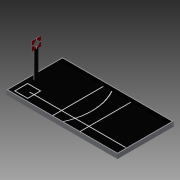
# Autodesk Inventor part: SEC 2014 Model1
Saved by Autodesk Inventor 2014 SP1 (Build 180222100, 222)
## iProperties
Created: 2014-01-13
Part Number: SEC 2014 Model1
Material: Generic
Document SubType Name: Modeling
Designer: Aaron
Density: 1 g/cm^3
Appearance: Default
Author: Aaron
Autodesk Inventor part; units mm, degrees
ref_plane "YZ Plane" through (0, 0, 0) normal (1, 0, 0) x (0, 1, 0)
ref_plane "XZ Plane" through (0, 0, 0) normal (0, 1, 0) x (-1, 0, 0)
ref_plane "XY Plane" through (0, 0, 0) normal (0, 0, 1) x (1, 0, 0)
sketch "Sketch1" plane through (0, 0, 0) normal (0, 1, 0) x (-1, 0, 0)
  line L0 (0, 0) -> (2463.8, 0)
  line L1 (2463.8, 0) -> (2463.8, -1244.6)
  line L2 (2463.8, -1244.6) -> (0, -1244.6)
  line L3 (0, -1244.6) -> (0, 0)
  dimension "d0" = 2463.8
  dimension "d1" = 1244.6
  constraints: 8 end point, 2 parallel, 1 horizontal, 1 perpendicular
  measures "d0" distance of L0.start L0.end
  measures "d1" distance of L2.end L0.start
extrude "Extrusion1" add sketch "Sketch1" along normal blind 12.7
sketch "Sketch2" plane through (0, 12.7, 0) normal (0, 1, 0) x (1, 0, 0)
  line L0 (-2463.8, 0) -> (0, 0) projected
  line L1 (0, 0) -> (0, 1244.6) projected
  line L2 (0, 1244.6) -> (-2463.8, 1244.6) projected
  line L3 (-2463.8, 1244.6) -> (-2463.8, 0) projected
  line L4 (-2444.75, 1225.55) -> (-19.05, 1225.55)
  line L5 (-19.05, 1225.55) -> (-19.05, 19.05)
  line L6 (-19.05, 19.05) -> (-2444.75, 19.05)
  line L7 (-2444.75, 19.05) -> (-2444.75, 1225.55)
  line L8 (-2463.8, 1244.6) -> (0, 1244.6)
  line L9 (0, 1244.6) -> (0, 0)
  line L10 (0, 0) -> (-2463.8, 0)
  line L11 (-2463.8, 0) -> (-2463.8, 1244.6)
  dimension "d4" = 19.05
  dimension "d5" = 19.05
  dimension "d6" = 19.05
  dimension "d7" = 19.05
  constraints: 16 end point, 4 parallel, 2 horizontal, 2 perpendicular
  measures "d4" distance from line of L2 L4.start
  measures "d5" distance from line of L3 L4.start
  measures "d6" distance from line of L1 L5.end
  measures "d7" distance from line of L0 L5.end
extrude "Extrusion2" add sketch "Sketch2" along normal blind 88.9
sketch "Sketch3" plane through (0, 12.7, 0) normal (0, 1, 0) x (1, 0, 0)
  line L0 (-19.05, 1225.55) -> (-2444.75, 1225.55) projected
  line L1 (-19.05, 19.05) -> (-19.05, 1225.55) projected
  line L2 (-19.05, 1225.55) -> (-2444.75, 1225.55) projected
  line L3 (-2444.75, 1225.55) -> (-2444.75, 19.05) projected
  line L4 (-2444.75, 19.05) -> (-19.05, 19.05) projected
  line L5 (-2463.8, 0) -> (0, 0) projected
  line L6 (-2463.8, 1244.6) -> (-2463.8, 0) projected
  line L7 (-19.05, 19.05) -> (-2444.75, 19.05) projected
  line L8 (-2444.75, 146.05) -> (-2139.95, 146.05)
  line L9 (-2139.95, 146.05) -> (-2139.95, 450.85)
  line L10 (-2139.95, 450.85) -> (-2444.75, 450.85)
  line L11 (-2444.75, 450.85) -> (-2444.75, 146.05)
  line L12 (-2425.7, 431.8) -> (-2159, 431.8)
  line L13 (-2159, 431.8) -> (-2159, 165.1)
  line L14 (-2159, 165.1) -> (-2425.7, 165.1)
  line L15 (-2425.7, 165.1) -> (-2425.7, 431.8)
  line L16 (-2248.2339, 307.975) -> (-114.6339, 307.975)
  line L17 (-114.6339, 307.975) -> (-114.6339, 288.925)
  line L18 (-114.6339, 288.925) -> (-2248.2339, 288.925)
  line L19 (-2248.2339, 288.925) -> (-2248.2339, 307.975)
  line L20 (-1549.4, 1225.55) -> (-1530.35, 1225.55)
  line L21 (-1530.35, 1225.55) -> (-1530.35, 19.05)
  line L22 (-1530.35, 19.05) -> (-1549.4, 19.05)
  line L23 (-1549.4, 19.05) -> (-1549.4, 1225.55)
  line L24 (-939.8, 1225.55) -> (-920.75, 1225.55)
  line L25 (-920.75, 1225.55) -> (-920.75, 19.05)
  line L26 (-920.75, 19.05) -> (-939.8, 19.05)
  line L27 (-939.8, 19.05) -> (-939.8, 1225.55)
  line L28 (-2444.75, 666.75) -> (-2425.7, 666.75)
  line L29 (-2425.7, 666.75) -> (-2425.7, 577.85)
  line L30 (-2425.7, 577.85) -> (-2444.75, 577.85)
  line L31 (-2444.75, 577.85) -> (-2444.75, 666.75)
  arc A0 (-1352.0706, 0) -> (-1341.2523, 1225.55) centre (-2425.7, 622.3) ccw
  arc A1 (-1374.1473, 0) -> (-1363.1042, 1225.55) centre (-2425.7, 622.3) ccw
  arc A2 (-1363.0943, 0) -> (-1352.1649, 19.05) centre (-2425.7, 622.3) ccw
  arc A3 (-1240.2679, 288.925) -> (-1235.075, 307.975) centre (-2425.7, 622.3) ccw
  line L32 (-1363.1042, 1225.55) -> (-1341.2523, 1225.55)
  line L33 (-1341.2523, 19.05) -> (-1363.1042, 19.05)
  point P0 (-2248.2339, 298.45)
  point P1 (-2444.75, 622.3)
  dimension "d10" = 127
  dimension "d11" = 304.8
  dimension "d12" = 304.8
  dimension "d13" = 19.05
  dimension "d14" = 19.05
  dimension "d15" = 266.7
  dimension "d16" = 266.7
  dimension "d17" = 9.525
  dimension "d18" = 2133.6
  dimension "d19" = 19.05
  dimension "d20" = 609.6
  dimension "d21" = 19.05
  dimension "d22" = 609.6
  dimension "d23" = 19.05
  dimension "d24" = 295.275
  dimension "d25" = 603.25
  dimension "d26" = 44.45
  dimension "d27" = 88.9
  dimension "d28" = 19.05
  dimension "d30" = 2481.8842
  dimension "d31" = 2443.7842
  constraints: 52 end point, 12 parallel, 11 point on line, 10 point on circle, 6 horizontal, 6 perpendicular, 4 centre point, 4 coincident, 2 midpoint, 1 collinear, 6 other
  measures "d10" distance of point (-2444.75, 19.05) L8.start
  measures "d11" distance of L8.start L8.end
  measures "d12" distance of L8.end L9.end
  measures "d13" distance from line of L10 L12.start
  measures "d14" distance from line of L11 L12.start
  measures "d15" distance of L12.start L12.end
  measures "d16" distance of L14.end L12.start
  measures "d17" distance of L16.start point (-2248.234, 298.45)
  measures "d18" distance of L16.start L16.end
  measures "d19" distance of L18.end L16.start
  measures "d20" distance from line of L13 L20.start
  measures "d21" distance between parallel lines of L21 L23
  measures "d22" distance of L24.start L20.start
  measures "d23" distance between parallel lines of L25 L27
  measures "d24" distance from line of A3.end L21
  measures "d25" distance from line of L0 point (-2444.75, 622.3)
  measures "d26" distance of point (-2444.75, 622.3) L28.start
  measures "d27" distance of L28.end L29.end
  measures "d28" distance of L28.start L28.end
  measures "d30" diameter of A0
  measures "d31" diameter of A1
extrude "Extrusion3" add sketch "Sketch3" along normal blind 1.5875 contours L25 L16 L27 L0 | L25 L18 L27 L16 | L16 L17 L18 L25 | L4 L27 L18 L25 | A0 L16 A1 L0 | L27 L18 A0 L16 | A0 L18 A3 L16 | L4 A1 L18 A0 | L21 L16 L23 L0 | A1 L18 L21 L16 | L16 A3 L18 A1 | A2 L5 A1 L4 | L21 L18 L23 L16 | L23 L18 L9 L16 | L21 L4 L23 L18 | L28 L29 L30 L3 | L16 L13 L12 L15 L14 L18 L9 L8 L3 L10 | L9 L18 L13 L16 | L13 L18 L19 L16
sketch "Sketch4" plane through (0, 12.7, 0) normal (0, 1, 0) x (1, 0, 0)
  line L0 (-1363.1042, 1225.55) -> (-1530.35, 1225.55) projected
  line L1 (-1530.35, 1225.55) -> (-1530.35, 307.975) projected
  line L2 (-2444.75, 1225.55) -> (-19.05, 1225.55) projected
  circle A0 centre (-1564.3323, 1073.15) radius 3.175
  circle A1 centre (-1564.3323, 1022.35) radius 3.175
  circle A2 centre (-1564.3323, 971.55) radius 3.175
  circle A3 centre (-1564.3323, 920.75) radius 3.175
  circle A4 centre (-1564.3323, 869.95) radius 3.175
  circle A5 centre (-1564.3323, 819.15) radius 3.175
  circle A6 centre (-1564.3323, 768.35) radius 3.175
  circle A7 centre (-1564.3323, 717.55) radius 3.175
  circle A8 centre (-1564.3323, 666.75) radius 3.175
  circle A9 centre (-1564.3323, 615.95) radius 3.175
  circle A10 centre (-1564.3323, 565.15) radius 3.175
  circle A11 centre (-1564.3323, 514.35) radius 3.175
  circle A12 centre (-1564.3323, 463.55) radius 3.175
  circle A13 centre (-1564.3323, 412.75) radius 3.175
  circle A14 centre (-1513.5323, 1073.15) radius 3.175
  circle A15 centre (-1513.5323, 1022.35) radius 3.175
  circle A16 centre (-1513.5323, 971.55) radius 3.175
  circle A17 centre (-1513.5323, 920.75) radius 3.175
  circle A18 centre (-1513.5323, 869.95) radius 3.175
  circle A19 centre (-1513.5323, 819.15) radius 3.175
  circle A20 centre (-1513.5323, 768.35) radius 3.175
  circle A21 centre (-1513.5323, 717.55) radius 3.175
  circle A22 centre (-1513.5323, 666.75) radius 3.175
  circle A23 centre (-1513.5323, 615.95) radius 3.175
  circle A24 centre (-1513.5323, 565.15) radius 3.175
  circle A25 centre (-1513.5323, 514.35) radius 3.175
  circle A26 centre (-1513.5323, 463.55) radius 3.175
  circle A27 centre (-1513.5323, 412.75) radius 3.175
  point P0 (0, 0)
  point P1 (-1353.5792, 1225.55)
  point P2 (-1378.9792, 1225.55)
  dimension "d38" = 152.4
  dimension "d41" = 50.8
  dimension "d42" = 6.35
  dimension "d45" = 50.8
  dimension "d50" = 6.35
  dimension "d53" = 50.8
  dimension "d58" = 9.525
  dimension "d59" = 25.4
  constraints: 28 centre point, 3 coincident, 2 point on line, 2 vertical, 52 other
  measures "d38" distance from line of L0 point (-1513.532, 1073.15)
  measures "d41" distance of point (-1564.332, 1073.15) point (-1564.332, 1022.35)
  measures "d42" diameter of A0
  measures "d45" distance of A0.centre A1.centre
  measures "d50" diameter of A14
  measures "d53" distance of A14.centre A15.centre
  measures "d58" distance of point (-1363.104, 1225.55) point (-1353.579, 1225.55)
  measures "d59" distance of point (-1353.579, 1225.55) point (-1378.979, 1225.55)
extrude "Extrusion4" cut sketch "Sketch4" against normal blind 25.4
sketch "Sketch5" plane through (0, 12.7, 0) normal (0, 1, 0) x (1, 0, 0)
  arc A0 (-1225.2263, 307.975) -> (-1341.2523, 1225.55) centre (-2425.7, 622.3) ccw projected
  line L0 (-1225.2263, 307.975) -> (-939.8, 307.975) projected
  line L1 (-939.8, 307.975) -> (-939.8, 1225.55) projected
  line L2 (-939.8, 1225.55) -> (-1341.2523, 1225.55) projected
  line L3 (-920.75, 1225.55) -> (-920.75, 307.975) projected
  line L4 (-920.75, 307.975) -> (-114.6339, 307.975) projected
  line L5 (-114.6339, 307.975) -> (-114.6339, 288.925) projected
  line L6 (-114.6339, 288.925) -> (-920.75, 288.925) projected
  line L7 (-920.75, 288.925) -> (-920.75, 19.05) projected
  line L8 (-920.75, 19.05) -> (-19.05, 19.05) projected
  line L9 (-19.05, 19.05) -> (-19.05, 1225.55) projected
  line L10 (-19.05, 1225.55) -> (-920.75, 1225.55) projected
  line L11 (-1341.2523, 19.05) -> (-1363.1042, 19.05) projected
  arc A1 (-1341.2523, 19.05) -> (-1230.3764, 288.925) centre (-2425.7, 622.3) ccw projected
  line L12 (-1230.3764, 288.925) -> (-939.8, 288.925) projected
  line L13 (-939.8, 288.925) -> (-939.8, 19.05) projected
  line L14 (-920.75, 19.05) -> (-939.8, 19.05) projected
  line L15 (-920.75, 19.05) -> (-920.75, 288.925) projected
  line L16 (-920.75, 288.925) -> (-114.6339, 288.925) projected
  line L17 (-114.6339, 288.925) -> (-114.6339, 307.975) projected
  line L18 (-114.6339, 307.975) -> (-920.75, 307.975) projected
  line L19 (-920.75, 307.975) -> (-920.75, 1225.55) projected
  line L20 (-939.8, 1225.55) -> (-920.75, 1225.55) projected
  line L21 (-939.8, 1225.55) -> (-939.8, 307.975) projected
  line L22 (-939.8, 307.975) -> (-1225.2263, 307.975) projected
  arc A2 (-1225.2263, 307.975) -> (-1341.2523, 1225.55) centre (-2425.7, 622.3) ccw projected
  line L23 (-1363.1042, 1225.55) -> (-1341.2523, 1225.55) projected
  arc A3 (-1244.929, 307.975) -> (-1363.1042, 1225.55) centre (-2425.7, 622.3) ccw projected
  line L24 (-1244.929, 307.975) -> (-1530.35, 307.975) projected
  line L25 (-1530.35, 307.975) -> (-1530.35, 1225.55) projected
  line L26 (-1549.4, 1225.55) -> (-1530.35, 1225.55) projected
  line L27 (-1549.4, 1225.55) -> (-1549.4, 307.975) projected
  line L28 (-1549.4, 307.975) -> (-2139.95, 307.975) projected
  line L29 (-2139.95, 307.975) -> (-2139.95, 450.85) projected
  line L30 (-2139.95, 450.85) -> (-2444.75, 450.85) projected
  line L31 (-2444.75, 146.05) -> (-2444.75, 450.85) projected
  line L32 (-2444.75, 146.05) -> (-2139.95, 146.05) projected
  line L33 (-2139.95, 146.05) -> (-2139.95, 288.925) projected
  line L34 (-2139.95, 288.925) -> (-1549.4, 288.925) projected
  line L35 (-1549.4, 288.925) -> (-1549.4, 19.05) projected
  line L36 (-1530.35, 19.05) -> (-1549.4, 19.05) projected
  line L37 (-1530.35, 19.05) -> (-1530.35, 288.925) projected
  line L38 (-1530.35, 288.925) -> (-1250.1655, 288.925) projected
  arc A4 (-1363.1042, 19.05) -> (-1250.1655, 288.925) centre (-2425.7, 622.3) ccw projected
  line L39 (-2159, 288.925) -> (-2159, 165.1) projected
  line L40 (-2159, 165.1) -> (-2425.7, 165.1) projected
  line L41 (-2425.7, 165.1) -> (-2425.7, 431.8) projected
  line L42 (-2425.7, 431.8) -> (-2159, 431.8) projected
  line L43 (-2159, 431.8) -> (-2159, 307.975) projected
  line L44 (-2159, 307.975) -> (-2248.2339, 307.975) projected
  line L45 (-2248.2339, 307.975) -> (-2248.2339, 288.925) projected
  line L46 (-2248.2339, 288.925) -> (-2159, 288.925) projected
  line L47 (-19.05, 1225.55) -> (-19.05, 19.05) projected
  line L48 (-19.05, 19.05) -> (-2444.75, 19.05) projected
  line L49 (-2444.75, 19.05) -> (-2444.75, 1225.55) projected
  line L50 (-2444.75, 1225.55) -> (-19.05, 1225.55) projected
  line L51 (0, 0) -> (0, 1244.6) projected
  line L52 (0, 1244.6) -> (-2463.8, 1244.6) projected
  line L53 (-2463.8, 1244.6) -> (-2463.8, 0) projected
  line L54 (-2463.8, 0) -> (0, 0) projected
  line L55 (-2444.75, 1225.55) -> (-19.05, 1225.55) projected
  arc A5 (-1352.1649, 19.05) -> (-1352.1649, 1225.55) centre (-2425.7, 622.3) ccw
  circle A6 centre (-1305.1845, 1073.15) radius 3.175
  circle A7 centre (-1286.4764, 1022.35) radius 3.175
  circle A8 centre (-1235.6764, 1022.35) radius 3.175
  circle A9 centre (-1270.2475, 971.55) radius 3.175
  circle A10 centre (-1219.4475, 971.55) radius 3.175
  circle A11 centre (-1256.3968, 920.75) radius 3.175
  circle A12 centre (-1205.5968, 920.75) radius 3.175
  circle A13 centre (-1244.8423, 869.95) radius 3.175
  circle A14 centre (-1194.0423, 869.95) radius 3.175
  circle A15 centre (-1235.5186, 819.15) radius 3.175
  circle A16 centre (-1184.7186, 819.15) radius 3.175
  circle A17 centre (-1254.3845, 1073.15) radius 3.175
  circle A18 centre (-1228.3746, 768.35) radius 3.175
  circle A19 centre (-1177.5746, 768.35) radius 3.175
  circle A20 centre (-1223.3722, 717.55) radius 3.175
  circle A21 centre (-1172.5722, 717.55) radius 3.175
  circle A22 centre (-1220.4854, 666.75) radius 3.175
  circle A23 centre (-1169.6854, 666.75) radius 3.175
  circle A24 centre (-1219.6993, 615.95) radius 3.175
  circle A25 centre (-1168.8993, 615.95) radius 3.175
  circle A26 centre (-1221.0098, 565.15) radius 3.175
  circle A27 centre (-1170.2098, 565.15) radius 3.175
  circle A28 centre (-1224.4236, 514.35) radius 3.175
  circle A29 centre (-1173.6236, 514.35) radius 3.175
  circle A30 centre (-1229.9585, 463.55) radius 3.175
  circle A31 centre (-1179.1585, 463.55) radius 3.175
  circle A32 centre (-1237.6434, 412.75) radius 3.175
  circle A33 centre (-1186.8434, 412.75) radius 3.175
  point P0 (-1279.7845, 1073.15)
  point P1 (-1261.0764, 1022.35)
  point P2 (-1244.8475, 971.55)
  point P3 (-1230.9968, 920.75)
  point P4 (-1219.4423, 869.95)
  point P5 (-1210.1186, 819.15)
  point P6 (-1202.9746, 768.35)
  point P7 (-1197.9722, 717.55)
  point P8 (-1195.0854, 666.75)
  point P9 (-1195.0854, 666.75)
  point P10 (-1194.2993, 615.95)
  point P11 (-1195.6098, 565.15)
  point P12 (-1199.0236, 514.35)
  point P13 (-1204.5585, 463.55)
  point P14 (-1212.2434, 412.75)
  point P15 (-1230.9968, 920.75)
  point P16 (-1219.4423, 869.95)
  dimension "d62" = 2462.8342
  dimension "d63" = 152.4
  dimension "d64" = 25.4
  dimension "d65" = 25.4
  dimension "d67" = 6.35
  dimension "d68" = 203.2
  dimension "d69" = 25.4
  dimension "d70" = 25.4
  dimension "d71" = 50.8
  dimension "d72" = 25.4
  dimension "d73" = 25.4
  dimension "d74" = 50.8
  dimension "d75" = 50.8
  dimension "d76" = 50.8
  dimension "d77" = 50.8
  dimension "d78" = 50.8
  dimension "d79" = 50.8
  dimension "d80" = 50.8
  dimension "d81" = 50.8
  dimension "d82" = 50.8
  dimension "d83" = 50.8
  dimension "d84" = 50.8
  dimension "d85" = 25.4
  dimension "d86" = 25.4
  dimension "d87" = 25.4
  dimension "d88" = 25.4
  dimension "d89" = 25.4
  dimension "d90" = 25.4
  dimension "d91" = 25.4
  dimension "d92" = 25.4
  dimension "d93" = 25.4
  dimension "d94" = 25.4
  dimension "d95" = 25.4
  dimension "d96" = 25.4
  dimension "d97" = 25.4
  dimension "d98" = 25.4
  dimension "d99" = 25.4
  dimension "d100" = 25.4
  dimension "d101" = 25.4
  dimension "d102" = 25.4
  dimension "d103" = 25.4
  dimension "d104" = 25.4
  dimension "d105" = 25.4
  dimension "d106" = 25.4
  dimension "d107" = 6.35
  dimension "d108" = 6.35
  dimension "d109" = 6.35
  dimension "d110" = 6.35
  dimension "d111" = 6.35
  dimension "d112" = 6.35
  dimension "d113" = 6.35
  dimension "d114" = 6.35
  dimension "d115" = 6.35
  dimension "d116" = 6.35
  dimension "d117" = 6.35
  dimension "d118" = 6.35
  dimension "d119" = 6.35
  dimension "d120" = 6.35
  dimension "d121" = 6.35
  dimension "d122" = 6.35
  dimension "d123" = 6.35
  dimension "d124" = 6.35
  dimension "d125" = 6.35
  dimension "d126" = 6.35
  dimension "d127" = 6.35
  constraints: 31 coincident, 28 centre point, 1 point on line, 21 other
  measures "d64" distance of point (-1305.184, 1073.15) point (-1279.784, 1073.15)
  measures "d65" distance of point (-1254.384, 1073.15) point (-1279.784, 1073.15)
  measures "d67" diameter of A6
  measures "d68" distance from line of L2 point (-1261.076, 1022.35)
  measures "d69" distance of point (-1261.076, 1022.35) point (-1286.476, 1022.35)
  measures "d70" distance of point (-1235.676, 1022.35) point (-1261.076, 1022.35)
  measures "d71" vertical distance of point (-1261.076, 1022.35) point (-1244.848, 971.55)
  measures "d72" distance of point (-1244.848, 971.55) point (-1270.248, 971.55)
  measures "d73" distance of point (-1244.848, 971.55) point (-1219.448, 971.55)
  measures "d74" vertical distance of point (-1244.848, 971.55) point (-1230.997, 920.75)
  measures "d75" vertical distance of point (-1230.997, 920.75) point (-1219.442, 869.95)
  measures "d76" vertical distance of point (-1219.442, 869.95) point (-1210.119, 819.15)
  measures "d77" vertical distance of point (-1202.975, 768.35) point (-1210.119, 819.15)
  measures "d78" vertical distance of point (-1202.975, 768.35) point (-1197.972, 717.55)
  measures "d79" vertical distance of point (-1197.972, 717.55) point (-1195.085, 666.75)
  measures "d80" vertical distance of point (-1195.085, 666.75) point (-1194.299, 615.95)
  measures "d81" vertical distance of point (-1194.299, 615.95) point (-1195.61, 565.15)
  measures "d82" vertical distance of point (-1195.61, 565.15) point (-1199.024, 514.35)
  measures "d83" vertical distance of point (-1199.024, 514.35) point (-1204.559, 463.55)
  measures "d84" vertical distance of point (-1212.243, 412.75) point (-1204.559, 463.55)
  measures "d85" distance of point (-1256.397, 920.75) point (-1230.997, 920.75)
  measures "d86" distance of point (-1205.597, 920.75) point (-1230.997, 920.75)
  measures "d87" distance of point (-1219.442, 869.95) point (-1244.842, 869.95)
  measures "d88" distance of point (-1194.042, 869.95) point (-1219.442, 869.95)
  measures "d89" distance of point (-1210.119, 819.15) point (-1235.519, 819.15)
  measures "d90" distance of point (-1184.719, 819.15) point (-1210.119, 819.15)
  measures "d91" distance of point (-1202.975, 768.35) point (-1228.375, 768.35)
  measures "d92" distance of point (-1177.575, 768.35) point (-1202.975, 768.35)
  measures "d93" distance of point (-1197.972, 717.55) point (-1223.372, 717.55)
  measures "d94" distance of point (-1172.572, 717.55) point (-1197.972, 717.55)
  measures "d95" distance of point (-1195.085, 666.75) point (-1220.485, 666.75)
  measures "d96" distance of point (-1169.685, 666.75) point (-1195.085, 666.75)
  measures "d97" distance of point (-1194.299, 615.95) point (-1219.699, 615.95)
  measures "d98" distance of point (-1168.899, 615.95) point (-1194.299, 615.95)
  measures "d99" distance of point (-1195.61, 565.15) point (-1221.01, 565.15)
  measures "d100" distance of point (-1170.21, 565.15) point (-1195.61, 565.15)
  measures "d101" distance of point (-1199.024, 514.35) point (-1224.424, 514.35)
  measures "d102" distance of point (-1173.624, 514.35) point (-1199.024, 514.35)
  measures "d103" distance of point (-1179.159, 463.55) point (-1204.559, 463.55)
  measures "d104" distance of point (-1204.559, 463.55) point (-1229.959, 463.55)
  measures "d105" distance of point (-1212.243, 412.75) point (-1237.643, 412.75)
  measures "d106" distance of point (-1186.843, 412.75) point (-1212.243, 412.75)
  measures "d107" diameter of A7
  measures "d108" diameter of A8
  measures "d109" diameter of A9
  measures "d110" diameter of A10
  measures "d111" diameter of A11
  measures "d112" diameter of A12
  measures "d113" diameter of A13
  measures "d114" diameter of A14
  measures "d115" diameter of A15
  measures "d116" diameter of A16
  measures "d117" diameter of A17
  measures "d118" diameter of A18
  measures "d119" diameter of A19
  measures "d120" diameter of A20
  measures "d121" diameter of A21
  measures "d122" diameter of A22
  measures "d123" diameter of A23
  measures "d124" diameter of A24
  measures "d125" diameter of A25
  measures "d126" diameter of A26
  measures "d127" diameter of A27
extrude "Extrusion5" cut sketch "Sketch5" against normal blind 25.4 contours A6 | A7 | A8 | A9 | A10 | A11 | A12 | A13 | A14 | A15 | A16 | A17 | A18 | A19 | A20 | A21 | A22 | A23 | A24 | A25 | A26 | A27 | A28 | A29 | A30 | A31 | A32 | A33
sketch "Sketch6" plane through (0, 12.7, 0) normal (0, 1, 0) x (1, 0, 0)
  line L0 (-939.8, 1225.55) -> (-939.8, 307.975) projected
  circle A0 centre (-1229.9585, 463.55) radius 3.175 projected
  circle A1 centre (-1221.0098, 565.15) radius 3.175 projected
  circle A2 centre (-1220.4854, 666.75) radius 3.175 projected
  circle A3 centre (-1228.3746, 768.35) radius 3.175 projected
  circle A4 centre (-1244.8423, 869.95) radius 3.175 projected
  circle A5 centre (-1270.2475, 971.55) radius 3.175 projected
  circle A6 centre (-1305.1845, 1073.15) radius 3.175 projected
  circle A7 centre (-1179.1585, 463.55) radius 3.175 projected
  circle A8 centre (-1170.2098, 565.15) radius 3.175 projected
  circle A9 centre (-1169.6854, 666.75) radius 3.175 projected
  circle A10 centre (-1177.5746, 768.35) radius 3.175 projected
  circle A11 centre (-1184.7186, 819.15) radius 3.175 projected
  circle A12 centre (-1205.5968, 920.75) radius 3.175 projected
  circle A13 centre (-1235.6764, 1022.35) radius 3.175 projected
  circle A14 centre (-1219.4475, 971.55) radius 3.175 projected
  circle A15 centre (-1194.0423, 869.95) radius 3.175 projected
  circle A16 centre (-1254.3845, 1073.15) radius 3.175 projected
  circle A17 centre (-1172.5722, 717.55) radius 3.175 projected
  circle A18 centre (-1168.8993, 615.95) radius 3.175 projected
  circle A19 centre (-1173.6236, 514.35) radius 3.175 projected
  circle A20 centre (-1186.8434, 412.75) radius 3.175 projected
  circle A21 centre (-1286.4764, 1022.35) radius 3.175 projected
  circle A22 centre (-1256.3968, 920.75) radius 3.175 projected
  circle A23 centre (-1235.5186, 819.15) radius 3.175 projected
  circle A24 centre (-1223.3722, 717.55) radius 3.175 projected
  circle A25 centre (-1219.6993, 615.95) radius 3.175 projected
  circle A26 centre (-1224.4236, 514.35) radius 3.175 projected
  circle A27 centre (-1237.6434, 412.75) radius 3.175 projected
  circle A28 centre (-1513.5323, 463.55) radius 3.175 projected
  circle A29 centre (-1513.5323, 565.15) radius 3.175 projected
  circle A30 centre (-1513.5323, 666.75) radius 3.175 projected
  circle A31 centre (-1513.5323, 768.35) radius 3.175 projected
  circle A32 centre (-1513.5323, 869.95) radius 3.175 projected
  circle A33 centre (-1513.5323, 971.55) radius 3.175 projected
  circle A34 centre (-1513.5323, 1073.15) radius 3.175 projected
  circle A35 centre (-1564.3323, 463.55) radius 3.175 projected
  circle A36 centre (-1564.3323, 565.15) radius 3.175 projected
  circle A37 centre (-1564.3323, 666.75) radius 3.175 projected
  circle A38 centre (-1564.3323, 768.35) radius 3.175 projected
  circle A39 centre (-1564.3323, 869.95) radius 3.175 projected
  circle A40 centre (-1564.3323, 971.55) radius 3.175 projected
  circle A41 centre (-1564.3323, 1073.15) radius 3.175 projected
  circle A42 centre (-1564.3323, 1022.35) radius 3.175 projected
  circle A43 centre (-1564.3323, 920.75) radius 3.175 projected
  circle A44 centre (-1564.3323, 819.15) radius 3.175 projected
  circle A45 centre (-1564.3323, 717.55) radius 3.175 projected
  circle A46 centre (-1564.3323, 615.95) radius 3.175 projected
  circle A47 centre (-1564.3323, 514.35) radius 3.175 projected
  circle A48 centre (-1564.3323, 412.75) radius 3.175 projected
  circle A49 centre (-1513.5323, 1022.35) radius 3.175 projected
  circle A50 centre (-1513.5323, 920.75) radius 3.175 projected
  circle A51 centre (-1513.5323, 819.15) radius 3.175 projected
  circle A52 centre (-1513.5323, 717.55) radius 3.175 projected
  circle A53 centre (-1513.5323, 615.95) radius 3.175 projected
  circle A54 centre (-1513.5323, 514.35) radius 3.175 projected
  circle A55 centre (-1513.5323, 412.75) radius 3.175 projected
  line L1 (0, 0) -> (-2463.8, 0) projected
  line L2 (-2463.8, 0) -> (-2463.8, 1244.6) projected
  line L3 (-2463.8, 1244.6) -> (0, 1244.6) projected
  line L4 (0, 1244.6) -> (0, 0) projected
  circle A56 centre (-955.675, 1073.15) radius 3.175
  circle A57 centre (-904.875, 1073.15) radius 3.175
  circle A58 centre (-955.675, 1022.35) radius 3.175
  circle A59 centre (-904.875, 1022.35) radius 3.175
  circle A60 centre (-955.675, 971.55) radius 3.175
  circle A61 centre (-904.875, 971.55) radius 3.175
  circle A62 centre (-955.675, 920.75) radius 3.175
  circle A63 centre (-904.875, 920.75) radius 3.175
  circle A64 centre (-955.675, 869.95) radius 3.175
  circle A65 centre (-904.875, 869.95) radius 3.175
  circle A66 centre (-955.675, 819.15) radius 3.175
  circle A67 centre (-904.875, 819.15) radius 3.175
  circle A68 centre (-955.675, 768.35) radius 3.175
  circle A69 centre (-904.875, 768.35) radius 3.175
  circle A70 centre (-955.675, 717.55) radius 3.175
  circle A71 centre (-904.875, 717.55) radius 3.175
  circle A72 centre (-955.675, 666.75) radius 3.175
  circle A73 centre (-904.875, 666.75) radius 3.175
  circle A74 centre (-955.675, 615.95) radius 3.175
  circle A75 centre (-904.875, 615.95) radius 3.175
  circle A76 centre (-955.675, 565.15) radius 3.175
  circle A77 centre (-904.875, 565.15) radius 3.175
  circle A78 centre (-955.675, 514.35) radius 3.175
  circle A79 centre (-904.875, 514.35) radius 3.175
  circle A80 centre (-955.675, 463.55) radius 3.175
  circle A81 centre (-904.875, 463.55) radius 3.175
  circle A82 centre (-955.675, 412.75) radius 3.175
  circle A83 centre (-904.875, 412.75) radius 3.175
  point P0 (-920.75, 1225.55)
  point P1 (-930.275, 1225.55)
  point P2 (-930.275, 1073.15)
  dimension "d136" = 9.525
  dimension "d137" = 152.4
  dimension "d138" = 25.4
  dimension "d139" = 25.4
  dimension "d140" = 6.35
  dimension "d141" = 6.35
  dimension "d144" = 50.8
  constraints: 28 centre point, 2 coincident, 1 vertical, 52 other
  measures "d136" distance of point (-920.75, 1225.55) point (-930.275, 1225.55)
  measures "d137" distance of point (-930.275, 1225.55) point (-930.275, 1073.15)
  measures "d138" distance of point (-955.675, 1073.15) point (-930.275, 1073.15)
  measures "d139" distance of point (-904.875, 1073.15) point (-930.275, 1073.15)
  measures "d140" diameter of A56
  measures "d141" diameter of A57
  measures "d144" distance of A56.centre A58.centre
extrude "Extrusion6" cut sketch "Sketch6" against normal blind 25.4 contours A56 | A57 | A58 | A59 | A60 | A61 | A62 | A63 | A64 | A65 | A66 | A67 | A68 | A69 | A70 | A71 | A72 | A73 | A74 | A75 | A76 | A77 | A78 | A79 | A80 | A81 | A82 | A83
sketch "Sketch7" plane through (0, 14.2875, 0) normal (0, 1, 0) x (1, 0, 0)
  line L0 (-2444.75, 577.85) -> (-2444.75, 666.75) projected
  line L1 (-2444.75, 577.85) -> (-2425.7, 577.85) projected
  line L2 (-2444.75, 666.75) -> (-2425.7, 666.75)
  line L3 (-2425.7, 666.75) -> (-2425.7, 577.85)
  line L4 (-2425.7, 577.85) -> (-2444.75, 577.85)
  line L5 (-2444.75, 577.85) -> (-2444.75, 666.75)
  point P0 (0, 0)
  constraints: 8 end point, 2 parallel, 1 horizontal, 1 perpendicular
extrude "Extrusion7" add sketch "Sketch7" along normal blind 608.0125
sketch "Sketch8" plane through (-2425.7, 12.7, -577.85) normal (1, 0, 0) x (0, 0, -1)
  line L0 (0, 609.6) -> (88.9, 609.6) projected
  line L1 (-57.15, 584.2) -> (146.05, 584.2)
  line L2 (146.05, 584.2) -> (146.05, 787.4)
  line L3 (146.05, 787.4) -> (-57.15, 787.4)
  line L4 (-57.15, 787.4) -> (-57.15, 584.2)
  point P0 (-577.85, -12.7)
  point P1 (44.45, 584.2)
  dimension "d153" = 25.4
  dimension "d154" = 101.6
  dimension "d155" = 203.2
  dimension "d156" = 203.2
  constraints: 8 end point, 2 parallel, 1 horizontal, 1 perpendicular
  measures "d153" distance from line of L0 point (44.45, 584.2)
  measures "d154" distance of L1.start point (44.45, 584.2)
  measures "d155" distance of L3.end L1.start
  measures "d156" distance of L2.end L3.end
extrude "Extrusion8" add sketch "Sketch8" along normal blind 6.35
sketch "Sketch9" plane through (-2419.35, 12.7, -577.85) normal (1, 0, 0) x (0, 0, -1)
  line L0 (-57.15, 584.2) -> (146.05, 584.2) projected
  line L1 (146.05, 584.2) -> (146.05, 787.4) projected
  line L2 (146.05, 787.4) -> (-57.15, 787.4) projected
  line L3 (-57.15, 787.4) -> (-57.15, 584.2) projected
  line L4 (34.925, 787.4) -> (53.975, 787.4)
  line L5 (53.975, 787.4) -> (53.975, 584.2)
  line L6 (53.975, 584.2) -> (34.925, 584.2)
  line L7 (34.925, 584.2) -> (34.925, 787.4)
  line L8 (146.05, 695.325) -> (-57.15, 695.325)
  line L9 (-57.15, 695.325) -> (-57.15, 676.275)
  line L10 (-57.15, 676.275) -> (146.05, 676.275)
  line L11 (146.05, 676.275) -> (146.05, 695.325)
  point P0 (-577.85, -12.7)
  point P1 (44.45, 787.4)
  point P2 (146.05, 685.8)
  dimension "d160" = 9.525
  dimension "d161" = 19.05
  dimension "d162" = 9.525
  dimension "d163" = 19.05
  constraints: 16 end point, 4 parallel, 4 point on line, 2 horizontal, 2 midpoint, 2 perpendicular
  measures "d160" distance of point (44.45, 787.4) L4.start
  measures "d161" distance between parallel lines of L5 L7
  measures "d162" distance of L8.start point (146.05, 685.8)
  measures "d163" distance between parallel lines of L10 L8
extrude "Extrusion9" add sketch "Sketch9" along normal blind 1.5875 contours L7 L10 L5 L0 | L3 L8 L7 L10 | L7 L8 L5 L10 | L5 L8 L1 L10 | L7 L2 L5 L8
sketch "Sketch10" plane through (-2417.7625, 12.7, -577.85) normal (1, 0, 0) x (0, 0, -1)
  circle A0 centre (44.45, 685.8) radius 63.5
  point P0 (-577.85, -12.7)
  dimension "d166" = 127
  constraints: 1 centre point
  measures "d166" diameter of A0
extrude "Extrusion10" cut sketch "Sketch10" against normal blind 25.4
body "Solid1"
